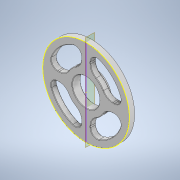
# Autodesk Inventor part: Zad 12
Saved by Autodesk Inventor 2020 (Build 240168000, 168)
## iProperties
Created: 2022-04-11
Part Number: Zad 12
Material: Ogólny
Document SubType Name: Modeling
Designer: 3IG
Density: 1 g/cm^3
Appearance: Domyślna
Author: 3IG
Autodesk Inventor part; units mm, degrees
ref_plane "YZ Plane" through (0, 0, 0) normal (1, 0, 0) x (0, 1, 0)
ref_plane "XZ Plane" through (0, 0, 0) normal (0, 1, 0) x (-1, 0, 0)
ref_plane "XY Plane" through (0, 0, 0) normal (0, 0, 1) x (1, 0, 0)
sketch "Szkic1" plane through (0, 0, 0) normal (0, 0, 1) x (1, 0, 0)
  circle A0 centre (0, 0) radius 15
  circle A1 centre (0, 0) radius 47.5
  dimension "d0" = 30
  dimension "d1" = 95
  constraints: 2 centre point, 2 coincident
  measures "d0" diameter of A0
  measures "d1" diameter of A1
extrude "Wyciągnięcie proste1" add sketch "Szkic1" along normal blind 6
sketch "Szkic2" plane through (0, 0, 6) normal (0, 0, 1) x (1, 0, 0)
  circle A0 centre (0, 0) radius 47.5 projected
  circle A1 centre (0, 0) radius 15 projected
  line L0 (-5, 29.4449) -> (-5, 31.277)
  line L1 (-29.4449, 5) -> (-31.277, 5)
  arc A2 (-11, 19.0526) -> (-19.0526, 11) centre (0, 0) ccw
  arc A3 (-11, 19.0526) -> (-5, 29.4449) centre (-17, 29.4449) ccw
  arc A4 (-29.4449, 5) -> (-19.0526, 11) centre (-29.4449, 17) ccw
  arc A5 (-14.5075, 37.8125) -> (-37.8125, 14.5075) centre (0, 0) ccw
  arc A6 (-5, 31.277) -> (-14.5075, 37.8125) centre (-12, 31.277) ccw
  arc A7 (-37.8125, 14.5075) -> (-31.277, 5) centre (-31.277, 12) ccw
  line L2 (-5, -29.4449) -> (-5, -31.277)
  line L3 (-29.4449, -5) -> (-31.277, -5)
  arc A8 (-19.0526, -11) -> (-11, -19.0526) centre (0, 0) ccw
  arc A9 (-37.8125, -14.5075) -> (-14.5075, -37.8125) centre (0, 0) ccw
  arc A10 (-19.0526, -11) -> (-29.4449, -5) centre (-29.4449, -17) ccw
  arc A11 (-5, -29.4449) -> (-11, -19.0526) centre (-17, -29.4449) ccw
  arc A12 (-14.5075, -37.8125) -> (-5, -31.277) centre (-12, -31.277) ccw
  arc A13 (-31.277, -5) -> (-37.8125, -14.5075) centre (-31.277, -12) ccw
  line L4 (5, -29.4449) -> (5, -31.277)
  line L5 (29.4449, -5) -> (31.277, -5)
  arc A14 (11, -19.0526) -> (19.0526, -11) centre (0, 0) ccw
  arc A15 (14.5075, -37.8125) -> (37.8125, -14.5075) centre (0, 0) ccw
  arc A16 (5, -31.277) -> (14.5075, -37.8125) centre (12, -31.277) ccw
  arc A17 (37.8125, -14.5075) -> (31.277, -5) centre (31.277, -12) ccw
  arc A18 (29.4449, -5) -> (19.0526, -11) centre (29.4449, -17) ccw
  arc A19 (11, -19.0526) -> (5, -29.4449) centre (17, -29.4449) ccw
  line L6 (31.277, 5) -> (29.4449, 5)
  line L7 (5, 31.277) -> (5, 29.4449)
  arc A20 (19.0526, 11) -> (11, 19.0526) centre (0, 0) ccw
  arc A21 (37.8125, 14.5075) -> (14.5075, 37.8125) centre (0, 0) ccw
  arc A22 (5, 29.4449) -> (11, 19.0526) centre (17, 29.4449) ccw
  arc A23 (19.0526, 11) -> (29.4449, 5) centre (29.4449, 17) ccw
  arc A24 (14.5075, 37.8125) -> (5, 31.277) centre (12, 31.277) ccw
  arc A25 (31.277, 5) -> (37.8125, 14.5075) centre (31.277, 12) ccw
  dimension "d21" = 12
  dimension "d22" = 7
  constraints: 48 point on circle, 32 tangent, 24 centre point, 16 end point, 8 equal radius, 4 horizontal, 4 vertical, 2 coincident
  measures "d21" radius of A22
  measures "d22" radius of A24
extrude "Wyciągnięcie proste2" cut sketch "Szkic2" against normal through all contours A3 A2 A4 L1 A7 A5 A6 L0 | L2 A12 A9 A13 L3 A10 A8 A11 | A19 A14 A18 L5 A17 A15 A16 L4 | L6 A23 A20 A22 L7 A24 A21 A25
sketch "Szkic3" plane through (0, 0, 0) normal (0, 0, -1) x (-1, 0, 0)
  circle A0 centre (0, 0) radius 22
  circle A1 centre (0, 0) radius 15
  constraints: 2 centre point, 2 coincident
extrude "Wyciągnięcie proste3" add sketch "Szkic3" along normal blind 3
sketch "Szkic7" plane through (0, 0, 6) normal (0, 0, 1) x (1, 0, 0)
  circle A0 centre (0, 0) radius 47.5 projected
  line L0 (0, -47.5) -> (0, 47.5)
  constraints: 2 end point, 2 point on circle, 1 vertical
ref_plane "Płaszczyzna konstrukcyjna4" through (0, -47.5, 6) normal (-1, 0, 0) x (0, 1, 0)
sketch "Szkic8" plane through (0, -47.5, 6) normal (-1, 0, 0) x (0, 1, 0)
  line L0 (69.5, 9) -> (25.5, 9) projected
  circle A0 centre (25.5, 9) radius 3
  line L1 (47.5, 6) -> (47.5, 9)
  line L2 (32.5, 9) -> (62.5, 9) projected
  point P0 (28.5, 9)
  point P1 (25.5, 6)
  dimension "d28" = 6
  constraints: 3 coincident, 2 end point, 2 point on circle, 1 centre point, 1 midpoint, 1 point on line
  measures "d28" diameter of A0
revolve "Obrót1" cut sketch "Szkic8" angle 360 about axis through (0, 0, 0) along (0, 0, -1)
chamfer "Faza1" distance 0.5 angle 45 60 edges at (15, 0, -3) (37.0455, 8.0347, 0) (28.6378, 28.6378, 0) (8.0347, 37.0455, 0) (5, 30.3609, 0) (6.6077, 23.4449, 0) (-15.5563, 15.5563, 0) (23.4449, 6.6077, 0) (30.3609, 5, 0) (37.0455, -8.0347, 0) (30.3609, -5, 0) (23.4449, -6.6077, 0) (6.6077, -23.4449, 0) (5, -30.3609, 0) (8.0347, -37.0455, 0) (28.6378, -28.6378, 0) (-6.6077, -23.4449, 0) (-23.4449, -6.6077, 0) (-30.3609, -5, 0) (-37.0455, -8.0347, 0) (-28.6378, -28.6378, 0) (-8.0347, -37.0455, 0) (-5, -30.3609, 0) (-5, 30.3609, 0) (-8.0347, 37.0455, 0) (-28.6378, 28.6378, 0) (-37.0455, 8.0347, 0) (-30.3609, 5, 0) (-23.4449, 6.6077, 0) (-6.6077, 23.4449, 0) (-6.6077, 23.4449, 6) (-15.5563, 15.5563, 6) (-23.4449, 6.6077, 6) (-30.3609, 5, 6) (-37.0455, 8.0347, 6) (-28.6378, 28.6378, 6) (-8.0347, 37.0455, 6) (-5, 30.3609, 6) (6.6077, 23.4449, 6) (5, 30.3609, 6) (8.0347, 37.0455, 6) (28.6378, 28.6378, 6) (37.0455, 8.0347, 6) (30.3609, 5, 6) (23.4449, 6.6077, 6) (23.4449, -6.6077, 6) (30.3609, -5, 6) (37.0455, -8.0347, 6) (28.6378, -28.6378, 6) (8.0347, -37.0455, 6) (5, -30.3609, 6) (6.6077, -23.4449, 6) (-6.6077, -23.4449, 6) (-5, -30.3609, 6) (-8.0347, -37.0455, 6) (-28.6378, -28.6378, 6) (-37.0455, -8.0347, 6) (-30.3609, -5, 6) (-23.4449, -6.6077, 6) (-15, 0, 6)
